Autodesk Fusion 360 part; units mm, degrees
note: some values were not read from the file. Set by a fixed rule: which sketch regions a step uses.
(part 2 of 3)
  constraint symmetric L0.start L152 L410.end
  constraint symmetric L5.start L152 L362.start
  constraint symmetric L6.end L152 L402.end
  constraint symmetric L9.end L152 L528.start
  constraint symmetric L7.end L152 L540.end
  constraint symmetric L18.start L152 L532.start
  constraint symmetric L21.start L152 L528.end
  constraint symmetric L19.start L152 L342.start
  constraint symmetric L9.start L152 L532.end
  constraint symmetric L1.end L152 L522.end
  constraint symmetric L11.end L152 L536.start
  constraint symmetric L1.start L152 L522.start
  constraint symmetric L20.end L152 L529.end
  constraint symmetric L4.start L152 L342.end
  constraint symmetric L4.end L152 L356.end
  constraint symmetric L2.start L152 L336.start
  constraint symmetric L25.start L152 L413.start
  constraint symmetric L24.start L152 L403.end
  constraint symmetric L24.end L152 L420.start
  constraint symmetric L25.end L152 L403.start
  constraint symmetric L29.start L152 L451.end
  constraint symmetric L28.start L152 L405.start
  constraint symmetric L28.end L152 L405.end
  constraint symmetric L29.end L152 L464.start
  constraint symmetric L33.start L152 L415.end
  constraint symmetric L32.start L152 L314.end
  constraint symmetric L32.end L152 L363.end
  constraint symmetric L33.end L152 L314.start
  constraint symmetric L42.start L152 L525.start
  constraint symmetric L49.start L152 L433.end
  constraint symmetric L39.start L152 L423.end
  constraint symmetric L61.start L152 L422.start
  constraint symmetric L57.start L152 L406.start
  constraint symmetric L52.start L152 L422.end
  constraint symmetric L60.end L152 L427.end
  constraint symmetric L52.end L152 L521.end
  constraint symmetric L66.end L152 L524.end
  constraint symmetric L37.end L152 L411.start
  constraint symmetric L47.start L152 L412.end
  constraint symmetric L40.end L152 L441.end
  constraint symmetric L38.end L152 L434.start
  constraint symmetric L40.start L152 L434.end
  constraint symmetric L38.start L152 L443.end
  constraint symmetric L53.end L152 L526.start
  constraint symmetric L48.start L152 L424.start
  constraint symmetric L48.end L152 L424.end
  constraint symmetric L42.end L152 L525.end
  constraint symmetric L50.end L152 L523.end
  constraint symmetric L37.start L152 L416.start
  constraint symmetric L45.start L152 L527.end
  constraint symmetric L58.start L152 L411.end
  constraint symmetric L41.end L152 L407.end
  constraint symmetric L54.end L152 L429.start
  constraint symmetric L41.start L152 L407.start
  constraint symmetric L56.start L152 L533.start
  constraint symmetric L69.end L152 L409.end
  constraint symmetric L36.end L152 L418.start
  constraint symmetric L36.start L152 L425.end
  constraint symmetric L46.end L152 L409.start
  constraint symmetric L44.start L152 L423.start
  constraint symmetric L62.start L152 L526.end
  constraint symmetric L57.end L152 L406.end
  constraint symmetric L39.end L152 L428.end
  constraint symmetric L59.end L152 L534.end
  constraint symmetric L72.start L152 L447.end
  constraint symmetric L73.end L152 L414.start
  constraint symmetric L74.start L152 L414.end
  constraint symmetric L72.end L152 L463.start
  constraint symmetric L79.end L152 L419.end
  constraint symmetric L107.start L152 L312.start
  constraint symmetric L88.start L152 L322.start
  constraint symmetric L91.end L152 L328.start
  constraint symmetric L77.start L152 L324.end
  constraint symmetric L77.end L152 L548.start
  constraint symmetric L78.start L152 L326.start
  constraint symmetric L76.end L152 L330.end
  constraint symmetric L82.end L152 L329.start
  constraint symmetric L84.start L152 L321.start
  constraint symmetric L95.end L152 L323.start
  constraint symmetric L110.end L152 L421.end
  constraint symmetric L83.start L152 L331.start
  constraint symmetric L89.start L152 L327.start
  constraint symmetric L86.end L152 L340.start
  constraint symmetric L98.end L152 L404.end
  constraint symmetric L108.start L152 L310.end
  constraint symmetric L94.end L152 L320.end
  constraint symmetric L113.start L152 L313.end
  constraint symmetric L94.start L152 L320.start
  constraint symmetric L95.start L152 L333.start
  constraint symmetric L81.start L152 L322.end
  constraint symmetric L103.start L152 L315.end
  constraint symmetric L108.end L152 L313.start
  constraint symmetric L82.start L152 L325.end
  constraint symmetric L89.end L152 L327.end
  constraint symmetric L102.end L152 L426.end
  constraint symmetric L84.end L152 L321.end
  constraint symmetric L98.start L152 L312.end
  constraint symmetric L104.start L152 L431.start
  constraint symmetric L103.end L152 L440.end
  constraint symmetric L83.end L152 L331.end
  constraint symmetric L92.end L152 L339.end
  constraint symmetric L105.end L152 L315.start
  constraint symmetric L105.start L152 L471.start
  constraint symmetric L81.end L152 L335.end
  constraint symmetric L92.start L152 L339.start
  constraint symmetric L113.end L152 L310.start
  constraint symmetric L80.start L152 L324.start
  constraint symmetric L76.start L152 L326.end
  constraint symmetric L118.end L152 L318.end
  constraint symmetric L130.end L152 L316.end
  constraint symmetric L147.start L152 L347.start
  constraint symmetric L118.start L152 L318.start
  constraint symmetric L119.end L152 L352.end
  constraint symmetric L134.start L152 L504.end
  constraint symmetric L116.start L152 L511.end
  constraint symmetric L136.start L152 L319.start
  constraint symmetric L136.end L152 L317.start
  constraint symmetric L129.start L152 L311.end
  constraint symmetric L126.start L152 L503.start
  constraint symmetric L130.start L152 L316.start
  constraint symmetric L128.start L152 L317.end
  constraint symmetric L124.start L152 L456.end
  constraint symmetric L124.end L152 L454.start
  constraint symmetric L139.end L152 L364.start
  constraint symmetric L122.start L152 L347.end
  constraint symmetric L119.start L152 L352.start
  constraint symmetric L133.start L152 L359.start
  constraint symmetric L135.end L152 L504.start
  constraint symmetric L116.end L152 L502.start
  constraint symmetric L134.end L152 L511.start
  constraint symmetric L127.start L152 L438.start
  constraint symmetric L143.start L152 L502.end
  constraint symmetric L117.start L152 L344.start
  constraint symmetric L117.end L152 L344.end
  constraint symmetric L121.start L152 L510.end
  constraint symmetric L132.start L152 L462.end
  constraint symmetric L121.end L152 L518.start
  constraint symmetric L123.end L152 L510.start
  constraint symmetric L123.start L152 L438.end
  constraint symmetric L128.end L152 L311.start
  constraint symmetric L133.end L152 L357.start
  constraint symmetric L120.end L152 L346.end
  constraint symmetric L120.start L152 L346.start
  constraint symmetric L125.start L152 L353.end
  constraint symmetric L152 L221.end L442.start
  constraint symmetric L152 L223.start L442.end
  constraint symmetric L152 L222.start L459.end
  constraint symmetric L152 L221.start L460.end
  constraint symmetric L152 L249.start L479.end
  constraint symmetric L152 L231.end L479.start
  constraint symmetric L152 L230.start L488.start
  constraint symmetric L152 L230.end L481.start
  constraint symmetric L152 L226.end L351.start
  constraint symmetric L152 L239.end L380.start
  constraint symmetric L152 L227.start L376.start
  constraint symmetric L152 L235.start L384.end
  constraint symmetric L152 L241.end L387.start
  constraint symmetric L152 L244.start L374.start
  constraint symmetric L152 L242.end L348.start
  constraint symmetric L152 L241.start L487.end
  constraint symmetric L152 L251.end L379.end
  constraint symmetric L152 L238.start L378.end
  constraint symmetric L152 L236.end L368.start
  constraint symmetric L152 L235.end L484.end
  constraint symmetric L152 L234.start L351.end
  constraint symmetric L152 L238.end L379.start
  constraint symmetric L152 L239.start L374.end
  constraint symmetric L152 L243.end L380.end
  constraint symmetric L152 L225.end L383.start
  constraint symmetric L152 L245.start L384.start
  constraint symmetric L152 L250.end L478.start
  constraint symmetric L152 L237.end L368.end
  constraint symmetric L152 L229.end L475.end
  constraint symmetric L152 L225.start L391.start
  constraint symmetric L152 L227.end L376.end
  constraint symmetric L152 L234.end L390.end
  constraint symmetric L152 L229.start L375.end
  constraint symmetric L152 L228.start L398.start
  constraint symmetric L152 L232.start L375.start
  constraint symmetric L152 L228.end L394.start
  constraint symmetric L152 L255.start L348.end
  constraint symmetric L152 L236.start L393.end
  constraint symmetric L152 L231.start L493.end
  constraint symmetric L152 L240.start L486.end
  constraint symmetric L152 L272.start L354.end
  constraint symmetric L152 L274.start L370.end
  constraint symmetric L152 L274.end L386.end
  constraint symmetric L152 L280.start L366.end
  constraint symmetric L152 L283.end L369.end
  constraint symmetric L152 L281.start L373.end
  constraint symmetric L152 L278.end L439.end
  constraint symmetric L152 L276.start L397.end
  constraint symmetric L152 L281.end L366.start
  constraint symmetric L152 L263.end L381.start
  constraint symmetric L152 L289.start L373.start
  constraint symmetric L152 L270.end L477.start
  constraint symmetric L152 L268.end L489.end
  constraint symmetric L152 L276.end L439.start
  constraint symmetric L152 L264.end L349.start
  constraint symmetric L152 L267.end L349.end
  constraint symmetric L152 L261.start L350.start
  constraint symmetric L152 L261.end L350.end
  constraint symmetric L152 L277.end L369.start
  constraint symmetric L152 L279.end L450.end
  constraint symmetric L152 L285.start L457.start
  constraint symmetric L152 L282.end L452.end
  constraint symmetric L152 L266.start L367.start
  constraint symmetric L152 L284.start L457.end
  constraint symmetric L152 L264.start L385.start
  constraint symmetric L152 L275.end L445.start
  constraint symmetric L152 L265.start L476.start
  constraint symmetric L152 L284.end L465.start
  constraint symmetric L152 L286.end L448.start
  constraint symmetric L152 L275.start L446.start
  constraint symmetric L152 L269.end L483.start
  constraint symmetric L152 L269.start L494.start
  constraint symmetric L152 L262.end L371.start
  constraint symmetric L152 L268.start L477.end
  constraint symmetric L152 L262.start L445.end
  constraint symmetric L152 L271.end L371.end
  constraint symmetric L152 P1 P8
  constraint symmetric L152 L298.start L455.start
  constraint symmetric L152 L298.end L455.end
  constraint symmetric L152 P2 P11
  constraint symmetric L152 L299.start L449.start
  constraint symmetric L152 L299.end L449.end
  constraint symmetric L152 P3 P10
  constraint symmetric L152 P4 P9
  constraint symmetric L152 P5 P7
  constraint symmetric L152 P6 P12
  constraint symmetric L152 L305.start L372.start
  constraint symmetric L152 L305.end L372.end
  constraint symmetric L152 L306.start L499.start
  constraint symmetric L152 L306.end L495.start
  constraint symmetric L152 L307.end L495.end
  constraint symmetric L152 L308.start L377.start
  constraint symmetric L152 L308.end L345.start
  constraint symmetric L152 L309.end L345.end
  constraint parallel L8 L550
  constraint perpendicular L550 L551
  constraint perpendicular L551 L552
  constraint tangent L552 A0
  constraint tangent A0 L553
  constraint parallel L285 L553
  constraint coincident L31 L552.end
  constraint coincident L290 A0.start
  constraint coincident L77 L550.end
  constraint symmetric L152 L550.start L554.start
  constraint symmetric L152 L550.end L554.end
  constraint symmetric L152 L551.end L555.end
  constraint symmetric L152 L552.end A1.start
  constraint symmetric L152 A0.start A1.end
  constraint symmetric L152 A0 A1
  constraint symmetric L152 L553.end L557.end
  constraint tangent L550 A2
  constraint tangent L554 A2
  constraint tangent A0 A3
  constraint coincident A3.end L558
  constraint tangent A3 L558
  constraint symmetric L152 A3.end A4.start
  constraint symmetric L152 A3 A4
  measures "d2" distance of L4.start L4.end
  measures "d3" distance of L20.end L4.end
  measures "d6" distance of L9.end L21.start
  measures "d7" distance of L18.start L21.start
  measures "d9" distance of L13.start L8.end
  measures "d10" distance of L13.start L2.start
  measures "d11" distance of L7.end L1.end
  measures "d12" distance of L7.end L11.end
  measures "d13" distance of L15 L17
  measures "d14" distance of L3.start L0.start
  measures "d15" distance of L0.end L0.start
  measures "d16" distance of L6.start L10.end
  measures "d17" distance of L6.start L6.end
  measures "d128" distance of L25.start L24.end
  measures "d129" distance of L25.start L25.end
  measures "d130" distance of L29.start L28.end
  measures "d131" distance of L29.start L29.end
  measures "d132" distance of L9 L11
  measures "d133" distance of L4 L13
  measures "d134" distance of L10 L21
  measures "d135" distance of L5 L22
  measures "d136" distance of L6 L24
  measures "d137" distance of L25 L28
  measures "d138" distance of L33.start L32.end
  measures "d139" distance of L33.start L33.end
  measures "d140" distance of L0 L32
  measures "d141" distance of L1 L8
  measures "d142" distance of L50.end L41.end
  measures "d143" distance of L50.end L45.start
  measures "d144" distance of L56.start L59.end
  measures "d145" distance of L42.start L56.start
  measures "d146" distance of L52.start L52.end
  measures "d147" distance of L52.end L54.end
  measures "d148" distance of L53.end L62.start
  measures "d149" distance of L48.start L62.start
  measures "d150" distance of L48 L52
  measures "d151" distance of L39.start L39.end
  measures "d152" distance of L49.start L39.end
  measures "d153" distance of L57.start L66.end
  measures "d154" distance of L57.start L57.end
  measures "d155" distance of L47.start L37.start
  measures "d156" distance of L37.end L37.start
  measures "d157" distance of L40.end L40.start
  measures "d158" distance of L40.end L38.start
  measures "d159" distance of L59 L62
  measures "d160" distance of L50 L54
  measures "d161" distance of L56 L66
  measures "d162" distance of L44 L45
  measures "d163" distance of L57 L58
  measures "d164" distance of L37 L51
  measures "d165" distance of L36.end L36.start
  measures "d166" distance of L36.end L46.end
  measures "d167" distance of L55 L71
  measures "d169" distance of L7 L67
  measures "d170" distance of L72.start L74.start
  measures "d171" distance of L72.start L72.end
  measures "d172" distance of L46 L75
  measures "d173" distance of L8 L61
  measures "d176" distance of L76.end L76.start
  measures "d177" distance of L79.end L76.end
  measures "d180" distance of L91.end L80.start
  measures "d181" distance of L77.start L80.start
  measures "d191" distance of L78 L80
  measures "d201" distance of L83.start L83.end
  measures "d202" distance of L89.start L83.end
  measures "d203" distance of L86.end L81.end
  measures "d204" distance of L88.start L86.end
  measures "d205" distance of L84.start L84.end
  measures "d206" distance of L82.start L84.end
  measures "d207" distance of L95.end L95.start
  measures "d208" distance of L95.end L94.start
  measures "d209" distance of L84 L94
  measures "d210" distance of L110.end L98.end
  measures "d211" distance of L107.start L110.end
  measures "d212" distance of L102.end L92.end
  measures "d213" distance of L102.end L104.start
  measures "d214" distance of L113.start L113.end
  measures "d215" distance of L108.start L113.end
  measures "d218" distance of L81 L100
  measures "d219" distance of L83 L93
  measures "d220" distance of L90 L92
  measures "d221" distance of L89 L98
  measures "d222" distance of L106 L114
  measures "d224" distance of L103.start L103.end
  measures "d225" distance of L103.end L105.start
  measures "d226" distance of L109 L111
  measures "d227" distance of L82 L96
  measures "d232" distance of L2 L95
  measures "d234" distance of L8 L85
  measures "d235" distance of L8 L91
  measures "d236" distance of L136.end L128.start
  measures "d237" distance of L136.start L136.end
  measures "d238" distance of L136.start L143.start
  measures "d239" distance of L129.start L128.end
  measures "d240" distance of L124.end L139.end
  measures "d241" distance of L119.end L119.start
  measures "d242" distance of L147.start L122.start
  measures "d245" distance of L135.end L121.end
  measures "d246" distance of L117.start L125.start
  measures "d247" distance of L134.start L135.end
  measures "d248" distance of L123.end L123.start
  measures "d249" distance of L127.start L123.start
  measures "d250" distance of L127 L142
  measures "d251" distance of L116.end L143.start
  measures "d252" distance of L138 L151
  measures "d254" distance of L116.start L134.end
  measures "d255" distance of L121.start L123.end
  measures "d256" distance of L129.start L126.start
  measures "d257" distance of L118.end L118.start
  measures "d258" distance of L79 L123
  measures "d261" distance of L155.end L155.start
  measures "d262" distance of L159.end L155.start
  measures "d263" distance of L159.end L159.start
  measures "d264" distance of L157.end L157.start
  measures "d265" distance of L181.start L179.start
  measures "d266" distance of L180.end L182.end
  measures "d267" distance of L180.start L179.end
  measures "d268" distance of L154.end L154.start
  measures "d269" distance of L174.end L171.start
  measures "d270" distance of L153.start L154.end
  measures "d271" distance of L162.end L156.end
  measures "d272" distance of L156.start L156.end
  measures "d273" distance of L156 L187
  measures "d274" distance of L159.start L161.end
  measures "d275" distance of L158 L163
  measures "d276" distance of L158.end L153.end
  measures "d277" distance of L162.end L168.end
  measures "d278" distance of L157.end L165.end
  measures "d279" distance of L167.start L167.end
  measures "d280" distance of L190.end L189.end
  measures "d281" distance of L190.end L191.end
  measures "d282" distance of L194.start L195.end
  measures "d283" distance of L193.start L194.start
  measures "d284" distance of L192 L196
  measures "d285" distance of L187 L194
  measures "d286" distance of P0 L196
  measures "d287" distance of L200.start L197.end
  measures "d288" distance of L200.end L200.start
  measures "d289" distance of L198.start L198.end
  measures "d290" distance of L198.end L199.start
  measures "d291" distance of L198 L203
  measures "d292" distance of L205.end L207.end
  measures "d293" distance of L206.start L207.end
  measures "d294" distance of L202 L206
  measures "d295" distance of L212.end L214.end
  measures "d296" distance of L216.start L214.end
  measures "d297" distance of L217.start L215.end
  measures "d298" distance of L217.end L217.start
  measures "d300" distance of L210.end L209.start
  measures "d301" distance of L209.end L209.start
  measures "d303" distance of L200 L212
  measures "d305" distance of L156 L197
  measures "d306" distance of L221.end L221.start
  measures "d307" distance of L221.end L223.start
  measures "d312" distance of L242.end L237.end
  measures "d313" distance of L236.end L237.end
  measures "d314" distance of L236.end L236.start
  measures "d315" distance of L238.start L255.start
  measures "d316" distance of L241.end L244.start
  measures "d317" distance of L243.end L250.end
  measures "d318" distance of L239.end L239.start
  measures "d319" distance of L230.end L225.start
  measures "d320" distance of L229.start L232.start
  measures "d321" distance of L225.end L225.start
  measures "d322" distance of L249.start L231.end
  measures "d323" distance of L231.end L231.start
  measures "d324" distance of L231 L245
  measures "d325" distance of L234.end L236.start
  measures "d326" distance of L248 L256
  measures "d327" distance of L226.end L234.start
  measures "d328" distance of L249.start L230.start
  measures "d329" distance of L238.start L238.end
  measures "d330" distance of L251.end L245.start
  measures "d375" distance of L272.start L267.end
  measures "d376" distance of L264.end L267.end
  measures "d377" distance of L264.end L264.start
  measures "d378" distance of L261.start L266.start
  measures "d379" distance of L274.start L274.end
  measures "d380" distance of L276.start L276.end
  measures "d381" distance of L283.end L277.end
  measures "d382" distance of L269.end L269.start
  measures "d383" distance of L284.start L284.end
  measures "d384" distance of L270.end L269.end
  measures "d385" distance of L262.end L262.start
  measures "d386" distance of L275.end L262.start
  measures "d387" distance of L289 L290
  measures "d388" distance of L264.start L265.start
  measures "d389" distance of L265 L268
  measures "d390" distance of L268.end L268.start
  measures "d391" distance of L262.end L271.end
  measures "d392" distance of L261.start L261.end
  measures "d393" distance of L263.end L289.start
  measures "d395" distance of origin L220
  measures "d397" angle of L190 L297
  measures "d398" angle of L77 L297
  measures "d399" angle of L30 L221
  measures "d401" distance of L221 L298
  measures "d402" distance of L30 P2
  measures "d403" distance of L29 P2
  measures "d404" distance of L298 P2
  measures "d405" distance of L223 L299
  measures "d406" distance of L77.end L189.end
  measures "d407" angle of L223 L233
  measures "d408" distance of L231 P5
  measures "d409" distance of L240 P5
  measures "d410" distance of L299 P5
  measures "d411" distance of L231 P6
  measures "d412" distance of L260 P6
  measures "d413" distance of L289 L305
  measures "d414" distance of P6 L305
  measures "d415" distance of L127 L306
  measures "d416" distance of L132 L307
  measures "d418" angle of L248 L289
  measures "d419" distance of L289 L308
  measures "d420" distance of L293 L309
  measures "d421" distance of L307 L308.end
  measures "d423" distance of L8 L550
  measures "d424" distance of L63 L551
  measures "d425" distance of L43 L552
extrude "Extrusion10" add sketch "Skizze1" along normal blind 3 makes body 1
sketch "Skizze5" plane through (0, 0, 0) normal (1, 0, 0) x (0, 1, 0)
  line L0 (0, 13.3887) -> (160, 20.3745)
  line L1 (0, 1.75) -> (0, 22.5)
  line L2 (1.75, 0) -> (22.5, 0)
  point P0 (14, 14)
  dimension "d440" = 2.5
  dimension "d441" = 160
  dimension "d450" = 14
  dimension "d451" = 14
  constraint coincident L0.start L1
  constraint coincident L0 P0
  measures "d440" angle of L0 L2
  measures "d441" distance of L0.end L1
  measures "d450" distance of L1 P0
  measures "d451" distance of L2 P0
ref_plane "Arbeitsebene1" through (0, 80, 16.8816) normal (0, 0.043619, -0.999048) x (0, 0.999048, 0.043619)
sketch "Skizze4" plane through (0, 0, 3) normal (0, 0, 1) x (-1, 0, 0)
  line L0 (88.256, -100.8256) -> (90.6871, -87.0383)
  line L1 (90.6871, -87.0383) -> (104.4744, -89.4694)
  line L2 (104.4744, -89.4694) -> (102.0433, -103.2567)
  line L3 (102.0433, -103.2567) -> (88.256, -100.8256)
  line L4 (123.6691, -90.3154) -> (121.238, -104.1027)
  line L5 (121.238, -104.1027) -> (107.4507, -101.6716)
  line L6 (107.4507, -101.6716) -> (109.8818, -87.8843)
  line L7 (109.8818, -87.8843) -> (123.6691, -90.3154)
  line L8 (87.3791, -105.7989) -> (101.1664, -108.23)
  line L9 (101.1664, -108.23) -> (98.7353, -122.0173)
  line L10 (98.7353, -122.0173) -> (84.948, -119.5862)
  line L11 (84.948, -119.5862) -> (87.3791, -105.7989)
  line L12 (100.8347, -139.1928) -> (103.2658, -125.4055)
  line L13 (103.2658, -125.4055) -> (117.0531, -127.8365)
  line L14 (117.0531, -127.8365) -> (114.622, -141.6239)
  line L15 (114.622, -141.6239) -> (100.8347, -139.1928)
  line L16 (97.8584, -126.9906) -> (95.4273, -140.7779)
  line L17 (95.4273, -140.7779) -> (81.64, -138.3468)
  line L18 (81.64, -138.3468) -> (84.0711, -124.5595)
  line L19 (84.0711, -124.5595) -> (97.8584, -126.9906)
  line L20 (-12.05, -83.05) -> (-26.05, -83.05)
  line L21 (-26.05, -83.05) -> (-26.05, -69.05)
  line L22 (-26.05, -69.05) -> (-12.05, -69.05)
  line L23 (-12.05, -69.05) -> (-12.05, -83.05)
  line L24 (147.396, -65.4579) -> (133.6087, -63.0268)
  line L25 (133.6087, -63.0268) -> (136.0398, -49.2395)
  line L26 (136.0398, -49.2395) -> (149.8271, -51.6706)
  line L27 (149.8271, -51.6706) -> (147.396, -65.4579)
  line L28 (29.7949, -103.261) -> (32.226, -89.4737)
  line L29 (32.226, -89.4737) -> (46.0133, -91.9047)
  line L30 (46.0133, -91.9047) -> (43.5823, -105.692)
  line L31 (43.5823, -105.692) -> (29.7949, -103.261)
  line L32 (69.0526, -100.0289) -> (82.8399, -102.46)
  line L33 (82.8399, -102.46) -> (80.4088, -116.2473)
  line L34 (80.4088, -116.2473) -> (66.6215, -113.8162)
  line L35 (66.6215, -113.8162) -> (69.0526, -100.0289)
  line L36 (47.3313, -113.5119) -> (61.1186, -115.9429)
  line L37 (61.1186, -115.9429) -> (58.6875, -129.7302)
  line L38 (58.6875, -129.7302) -> (44.9002, -127.2992)
  line L39 (44.9002, -127.2992) -> (47.3313, -113.5119)
  line L40 (42.7053, -110.6653) -> (40.2743, -124.4526)
  line L41 (40.2743, -124.4526) -> (26.4869, -122.0216)
  line L42 (26.4869, -122.0216) -> (28.918, -108.2342)
  line L43 (28.918, -108.2342) -> (42.7053, -110.6653)
  line L44 (65.7446, -118.7895) -> (79.5319, -121.2205)
  line L45 (79.5319, -121.2205) -> (77.1008, -135.0079)
  line L46 (77.1008, -135.0079) -> (63.3135, -132.5768)
  line L47 (63.3135, -132.5768) -> (65.7446, -118.7895)
  line L48 (48.2082, -108.5386) -> (50.6393, -94.7513)
  line L49 (50.6393, -94.7513) -> (64.4266, -97.1823)
  line L50 (64.4266, -97.1823) -> (61.9955, -110.9697)
  line L51 (61.9955, -110.9697) -> (48.2082, -108.5386)
  line L52 (72.3606, -81.2683) -> (86.1479, -83.6994)
  line L53 (86.1479, -83.6994) -> (83.7168, -97.4867)
  line L54 (83.7168, -97.4867) -> (69.9295, -95.0556)
  line L55 (69.9295, -95.0556) -> (72.3606, -81.2683)
  line L56 (53.9473, -75.9907) -> (67.7346, -78.4218)
  line L57 (67.7346, -78.4218) -> (65.3035, -92.2091)
  line L58 (65.3035, -92.2091) -> (51.5162, -89.778)
  line L59 (51.5162, -89.778) -> (53.9473, -75.9907)
  line L60 (57.2553, -57.2301) -> (71.0426, -59.6612)
  line L61 (71.0426, -59.6612) -> (68.6115, -73.4485)
  line L62 (68.6115, -73.4485) -> (54.8242, -71.0174)
  line L63 (54.8242, -71.0174) -> (57.2553, -57.2301)
  line L64 (75.6686, -62.5077) -> (89.4559, -64.9388)
  line L65 (89.4559, -64.9388) -> (87.0248, -78.7261)
  line L66 (87.0248, -78.7261) -> (73.2375, -76.295)
  line L67 (73.2375, -76.295) -> (75.6686, -62.5077)
  line L68 (46.8808, -85.6605) -> (40.6913, -84.5691)
  line L69 (40.6913, -84.5691) -> (40.548, -85.3816)
  line L70 (40.548, -85.3816) -> (37.8053, -84.898)
  line L71 (37.8053, -84.898) -> (37.9486, -84.0855)
  line L72 (37.9486, -84.0855) -> (34.7677, -83.5246)
  line L73 (34.7677, -83.5246) -> (35.9398, -76.8772)
  line L74 (35.9398, -76.8772) -> (39.1207, -77.4381)
  line L75 (39.1207, -77.4381) -> (39.3855, -75.9362)
  line L76 (39.3855, -75.9362) -> (34.7569, -75.1201)
  line L77 (34.7569, -75.1201) -> (37.188, -61.3328)
  line L78 (37.188, -61.3328) -> (41.8166, -62.1489)
  line L79 (41.8166, -62.1489) -> (42.0814, -60.6471)
  line L80 (42.0814, -60.6471) -> (38.9005, -60.0862)
  line L81 (38.9005, -60.0862) -> (40.0726, -53.4388)
  line L82 (40.0726, -53.4388) -> (43.2536, -53.9996)
  line L83 (43.2536, -53.9996) -> (43.3968, -53.1872)
  line L84 (43.3968, -53.1872) -> (46.1395, -53.6708)
  line L85 (46.1395, -53.6708) -> (45.9962, -54.4833)
  line L86 (45.9962, -54.4833) -> (52.1858, -55.5746)
  line L87 (52.1858, -55.5746) -> (51.8862, -57.2734)
  line L88 (51.8862, -57.2734) -> (53.068, -57.4818)
  line L89 (53.068, -57.4818) -> (52.4949, -60.7317)
  line L90 (52.4949, -60.7317) -> (51.3132, -60.5233)
  line L91 (51.3132, -60.5233) -> (51.0136, -62.2221)
  line L92 (51.0136, -62.2221) -> (46.6115, -61.4459)
  line L93 (46.6115, -61.4459) -> (46.3467, -62.9477)
  line L94 (46.3467, -62.9477) -> (50.9753, -63.7639)
  line L95 (50.9753, -63.7639) -> (48.5442, -77.5512)
  line L96 (48.5442, -77.5512) -> (43.9157, -76.735)
  line L97 (43.9157, -76.735) -> (43.6508, -78.2368)
  line L98 (43.6508, -78.2368) -> (48.0529, -79.0131)
  line L99 (48.0529, -79.0131) -> (47.7534, -80.7118)
  line L100 (47.7534, -80.7118) -> (48.9352, -80.9202)
  line L101 (48.9352, -80.9202) -> (48.3621, -84.1701)
  line L102 (48.3621, -84.1701) -> (47.1803, -83.9617)
  line L103 (47.1803, -83.9617) -> (46.8808, -85.6605)
  line L104 (12.05, -69.05) -> (26.05, -69.05)
  line L105 (26.05, -69.05) -> (26.05, -83.05)
  line L106 (26.05, -83.05) -> (12.05, -83.05)
  line L107 (12.05, -83.05) -> (12.05, -69.05)
  line L108 (26.05, -50) -> (26.05, -64)
  line L109 (26.05, -64) -> (12.05, -64)
  line L110 (12.05, -64) -> (12.05, -50)
  line L111 (12.05, -50) -> (26.05, -50)
  line L112 (-12.05, -50) -> (-12.05, -64)
  line L113 (-12.05, -64) -> (-26.05, -64)
  line L114 (-26.05, -64) -> (-26.05, -50)
  line L115 (-26.05, -50) -> (-12.05, -50)
  line L116 (-7, -50) -> (7, -50)
  line L117 (7, -50) -> (7, -64)
  line L118 (7, -64) -> (-7, -64)
  line L119 (-7, -64) -> (-7, -50)
  line L120 (100.3693, -38.0507) -> (113.525, -42.8389)
  line L121 (113.525, -42.8389) -> (108.7367, -55.9946)
  line L122 (108.7367, -55.9946) -> (95.581, -51.2064)
  line L123 (95.581, -51.2064) -> (100.3693, -38.0507)
  line L124 (69.7598, -36.262) -> (72.1098, -32.1916)
  line L125 (72.1098, -32.1916) -> (84.2342, -39.1916)
  line L126 (84.2342, -39.1916) -> (81.8842, -43.262)
  line L127 (81.8842, -43.262) -> (83.2049, -44.0245)
  line L128 (83.2049, -44.0245) -> (84.8199, -41.2272)
  line L129 (84.8199, -41.2272) -> (90.6655, -44.6022)
  line L130 (90.6655, -44.6022) -> (89.0505, -47.3995)
  line L131 (89.0505, -47.3995) -> (89.765, -47.812)
  line L132 (89.765, -47.812) -> (88.3725, -50.2238)
  line L133 (88.3725, -50.2238) -> (87.658, -49.8113)
  line L134 (87.658, -49.8113) -> (84.5155, -55.2543)
  line L135 (84.5155, -55.2543) -> (83.0216, -54.3918)
  line L136 (83.0216, -54.3918) -> (82.4216, -55.431)
  line L137 (82.4216, -55.431) -> (79.5638, -53.781)
  line L138 (79.5638, -53.781) -> (80.1638, -52.7418)
  line L139 (80.1638, -52.7418) -> (78.6699, -51.8793)
  line L140 (78.6699, -51.8793) -> (80.9049, -48.0082)
  line L141 (80.9049, -48.0082) -> (79.5842, -47.2457)
  line L142 (79.5842, -47.2457) -> (77.2342, -51.316)
  line L143 (77.2342, -51.316) -> (65.1098, -44.316)
  line L144 (65.1098, -44.316) -> (67.4598, -40.2457)
  line L145 (67.4598, -40.2457) -> (66.1391, -39.4832)
  line L146 (66.1391, -39.4832) -> (63.9041, -43.3543)
  line L147 (63.9041, -43.3543) -> (62.4102, -42.4918)
  line L148 (62.4102, -42.4918) -> (61.8102, -43.531)
  line L149 (61.8102, -43.531) -> (58.9523, -41.881)
  line L150 (58.9523, -41.881) -> (59.5523, -40.8418)
  line L151 (59.5523, -40.8418) -> (58.0585, -39.9793)
  line L152 (58.0585, -39.9793) -> (61.201, -34.5363)
  line L153 (61.201, -34.5363) -> (60.4865, -34.1238)
  line L154 (60.4865, -34.1238) -> (61.879, -31.712)
  line L155 (61.879, -31.712) -> (62.5935, -32.1245)
  line L156 (62.5935, -32.1245) -> (64.2085, -29.3272)
  line L157 (64.2085, -29.3272) -> (70.0541, -32.7022)
  line L158 (70.0541, -32.7022) -> (68.4391, -35.4995)
  line L159 (68.4391, -35.4995) -> (69.7598, -36.262)
  line L160 (-65.7446, -118.7895) -> (-63.3135, -132.5768)
  line L161 (-63.3135, -132.5768) -> (-77.1008, -135.0079)
  line L162 (-77.1008, -135.0079) -> (-79.5319, -121.2205)
  line L163 (-79.5319, -121.2205) -> (-65.7446, -118.7895)
  line L164 (-81.64, -138.3468) -> (-95.4273, -140.7779)
  line L165 (-95.4273, -140.7779) -> (-97.8584, -126.9906)
  line L166 (-97.8584, -126.9906) -> (-84.0711, -124.5595)
  line L167 (-84.0711, -124.5595) -> (-81.64, -138.3468)
  line L168 (15.275, -92.8) -> (16.1, -92.8)
  line L169 (16.1, -92.8) -> (16.1, -95.585)
  line L170 (16.1, -95.585) -> (15.275, -95.585)
  line L171 (15.275, -95.585) -> (15.275, -101.87)
  line L172 (15.275, -101.87) -> (13.55, -101.87)
  line L173 (13.55, -101.87) -> (13.55, -103.07)
  line L174 (13.55, -103.07) -> (10.25, -103.07)
  line L175 (10.25, -103.07) -> (10.25, -101.87)
  line L176 (10.25, -101.87) -> (8.525, -101.87)
  line L177 (8.525, -101.87) -> (8.525, -97.4)
  line L178 (8.525, -97.4) -> (7, -97.4)
  line L179 (7, -97.4) -> (7, -102.1)
  line L180 (7, -102.1) -> (-7, -102.1)
  line L181 (-7, -102.1) -> (-7, -97.4)
  line L182 (-7, -97.4) -> (-8.525, -97.4)
  line L183 (-8.525, -97.4) -> (-8.525, -101.87)
  line L184 (-8.525, -101.87) -> (-10.25, -101.87)
  line L185 (-10.25, -101.87) -> (-10.25, -103.07)
  line L186 (-10.25, -103.07) -> (-13.55, -103.07)
  line L187 (-13.55, -103.07) -> (-13.55, -101.87)
  line L188 (-13.55, -101.87) -> (-15.275, -101.87)
  line L189 (-15.275, -101.87) -> (-15.275, -95.585)
  line L190 (-15.275, -95.585) -> (-16.1, -95.585)
  line L191 (-16.1, -95.585) -> (-16.1, -92.8)
  line L192 (-16.1, -92.8) -> (-15.275, -92.8)
  line L193 (-15.275, -92.8) -> (-15.275, -89.57)
  line L194 (-15.275, -89.57) -> (-8.525, -89.57)
  line L195 (-8.525, -89.57) -> (-8.525, -92.8)
  line L196 (-8.525, -92.8) -> (-7, -92.8)
  line L197 (-7, -92.8) -> (-7, -88.1)
  line L198 (-7, -88.1) -> (7, -88.1)
  line L199 (7, -88.1) -> (7, -92.8)
  line L200 (7, -92.8) -> (8.525, -92.8)
  line L201 (8.525, -92.8) -> (8.525, -89.57)
  line L202 (8.525, -89.57) -> (15.275, -89.57)
  line L203 (15.275, -89.57) -> (15.275, -92.8)
  line L204 (-7, -83.05) -> (-7, -69.05)
  line L205 (-7, -69.05) -> (7, -69.05)
  line L206 (7, -69.05) -> (7, -83.05)
  line L207 (7, -83.05) -> (-7, -83.05)
  line L208 (-2.525, -107.15) -> (-2.525, -121.15)
  line L209 (-2.525, -121.15) -> (-16.525, -121.15)
  line L210 (-16.525, -121.15) -> (-16.525, -107.15)
  line L211 (-16.525, -107.15) -> (-2.525, -107.15)
  line L212 (2.525, -121.15) -> (2.525, -107.15)
  line L213 (2.525, -107.15) -> (16.525, -107.15)
  line L214 (16.525, -107.15) -> (16.525, -121.15)
  line L215 (16.525, -121.15) -> (2.525, -121.15)
  line L216 (-46.0133, -91.9047) -> (-32.226, -89.4737)
  line L217 (-32.226, -89.4737) -> (-29.7949, -103.261)
  line L218 (-29.7949, -103.261) -> (-43.5823, -105.692)
  line L219 (-43.5823, -105.692) -> (-46.0133, -91.9047)
  line L220 (-113.1898, -69.1237) -> (-110.7587, -82.911)
  line L221 (-110.7587, -82.911) -> (-124.546, -85.3421)
  line L222 (-124.546, -85.3421) -> (-126.9771, -71.5548)
  line L223 (-126.9771, -71.5548) -> (-113.1898, -69.1237)
  line L224 (-130.3007, -81.7874) -> (-144.088, -84.2185)
  line L225 (-144.088, -84.2185) -> (-146.5191, -70.4311)
  line L226 (-146.5191, -70.4311) -> (-132.7318, -68.0001)
  line L227 (-132.7318, -68.0001) -> (-130.3007, -81.7874)
  line L228 (-149.0613, -85.0954) -> (-162.8486, -87.5265)
  line L229 (-162.8486, -87.5265) -> (-165.2797, -73.7391)
  line L230 (-165.2797, -73.7391) -> (-151.4924, -71.3081)
  line L231 (-151.4924, -71.3081) -> (-149.0613, -85.0954)
  line L232 (-143.2111, -89.1917) -> (-129.4238, -86.7607)
  line L233 (-129.4238, -86.7607) -> (-126.9927, -100.548)
  line L234 (-126.9927, -100.548) -> (-140.78, -102.979)
  line L235 (-140.78, -102.979) -> (-143.2111, -89.1917)
  line L236 (-168.5877, -54.9786) -> (-154.8004, -52.5475)
  line L237 (-154.8004, -52.5475) -> (-152.3693, -66.3348)
  line L238 (-152.3693, -66.3348) -> (-166.1566, -68.7659)
  line L239 (-166.1566, -68.7659) -> (-168.5877, -54.9786)
  line L240 (-147.396, -65.4579) -> (-149.8271, -51.6706)
  line L241 (-149.8271, -51.6706) -> (-136.0398, -49.2395)
  line L242 (-136.0398, -49.2395) -> (-133.6087, -63.0268)
  line L243 (-133.6087, -63.0268) -> (-147.396, -65.4579)
  line L244 (34.0551, -40.0943) -> (34.5854, -39.4624)
  line L245 (34.5854, -39.4624) -> (32.1111, -37.3861)
  line L246 (32.1111, -37.3861) -> (36.4499, -32.2153)
  line L247 (36.4499, -32.2153) -> (38.9242, -34.2916)
  line L248 (38.9242, -34.2916) -> (39.9045, -33.1233)
  line L249 (39.9045, -33.1233) -> (36.3041, -30.1022)
  line L250 (36.3041, -30.1022) -> (45.3031, -19.3776)
  line L251 (45.3031, -19.3776) -> (48.9035, -22.3987)
  line L252 (48.9035, -22.3987) -> (49.8838, -21.2305)
  line L253 (49.8838, -21.2305) -> (47.4094, -19.1543)
  line L254 (47.4094, -19.1543) -> (51.7483, -13.9835)
  line L255 (51.7483, -13.9835) -> (54.2226, -16.0597)
  line L256 (54.2226, -16.0597) -> (54.7529, -15.4277)
  line L257 (54.7529, -15.4277) -> (56.8863, -17.2179)
  line L258 (56.8863, -17.2179) -> (56.356, -17.8499)
  line L259 (56.356, -17.8499) -> (61.1706, -21.8898)
  line L260 (61.1706, -21.8898) -> (60.0618, -23.2112)
  line L261 (60.0618, -23.2112) -> (60.9811, -23.9825)
  line L262 (60.9811, -23.9825) -> (58.8599, -26.5105)
  line L263 (58.8599, -26.5105) -> (57.9406, -25.7392)
  line L264 (57.9406, -25.7392) -> (56.8318, -27.0606)
  line L265 (56.8318, -27.0606) -> (53.4076, -24.1873)
  line L266 (53.4076, -24.1873) -> (52.4273, -25.3555)
  line L267 (52.4273, -25.3555) -> (56.0277, -28.3766)
  line L268 (56.0277, -28.3766) -> (47.0287, -39.1013)
  line L269 (47.0287, -39.1013) -> (43.4283, -36.0802)
  line L270 (43.4283, -36.0802) -> (42.448, -37.2484)
  line L271 (42.448, -37.2484) -> (45.8723, -40.1216)
  line L272 (45.8723, -40.1216) -> (44.7635, -41.4431)
  line L273 (44.7635, -41.4431) -> (45.6827, -42.2144)
  line L274 (45.6827, -42.2144) -> (43.5615, -44.7424)
  line L275 (43.5615, -44.7424) -> (42.6423, -43.971)
  line L276 (42.6423, -43.971) -> (41.5335, -45.2924)
  line L277 (41.5335, -45.2924) -> (36.7189, -41.2525)
  line L278 (36.7189, -41.2525) -> (36.1886, -41.8845)
  line L279 (36.1886, -41.8845) -> (34.0551, -40.0943)
  line L280 (-66.6215, -113.8162) -> (-80.4088, -116.2473)
  line L281 (-80.4088, -116.2473) -> (-82.8399, -102.46)
  line L282 (-82.8399, -102.46) -> (-69.0526, -100.0289)
  line L283 (-69.0526, -100.0289) -> (-66.6215, -113.8162)
  line L284 (-61.1186, -115.9429) -> (-47.3313, -113.5119)
  line L285 (-47.3313, -113.5119) -> (-44.9002, -127.2992)
  line L286 (-44.9002, -127.2992) -> (-58.6875, -129.7302)
  line L287 (-58.6875, -129.7302) -> (-61.1186, -115.9429)
  line L288 (-48.2082, -108.5386) -> (-61.9955, -110.9697)
  line L289 (-61.9955, -110.9697) -> (-64.4266, -97.1823)
  line L290 (-64.4266, -97.1823) -> (-50.6393, -94.7513)
  line L291 (-50.6393, -94.7513) -> (-48.2082, -108.5386)
  line L292 (-127.854, -66.5815) -> (-130.2851, -52.7942)
  line L293 (-130.2851, -52.7942) -> (-116.4978, -50.3631)
  line L294 (-116.4978, -50.3631) -> (-114.0667, -64.1504)
  line L295 (-114.0667, -64.1504) -> (-127.854, -66.5815)
  line L296 (-95.581, -51.2064) -> (-108.7367, -55.9946)
  line L297 (-108.7367, -55.9946) -> (-113.525, -42.8389)
  line L298 (-113.525, -42.8389) -> (-100.3693, -38.0507)
  line L299 (-100.3693, -38.0507) -> (-95.581, -51.2064)
  line L300 (-68.6115, -73.4485) -> (-71.0426, -59.6612)
  line L301 (-71.0426, -59.6612) -> (-57.2553, -57.2301)
  line L302 (-57.2553, -57.2301) -> (-54.8242, -71.0174)
  line L303 (-54.8242, -71.0174) -> (-68.6115, -73.4485)
  line L304 (-81.8842, -43.262) -> (-84.2342, -39.1916)
  line L305 (-84.2342, -39.1916) -> (-72.1098, -32.1916)
  line L306 (-72.1098, -32.1916) -> (-69.7598, -36.262)
  line L307 (-69.7598, -36.262) -> (-68.4391, -35.4995)
  line L308 (-68.4391, -35.4995) -> (-70.0541, -32.7022)
  line L309 (-70.0541, -32.7022) -> (-64.2085, -29.3272)
  line L310 (-64.2085, -29.3272) -> (-62.5935, -32.1245)
  line L311 (-62.5935, -32.1245) -> (-61.879, -31.712)
  line L312 (-61.879, -31.712) -> (-60.4865, -34.1238)
  line L313 (-60.4865, -34.1238) -> (-61.201, -34.5363)
  line L314 (-61.201, -34.5363) -> (-58.0585, -39.9793)
  line L315 (-58.0585, -39.9793) -> (-59.5523, -40.8418)
  line L316 (-59.5523, -40.8418) -> (-58.9523, -41.881)
  line L317 (-58.9523, -41.881) -> (-61.8102, -43.531)
  line L318 (-61.8102, -43.531) -> (-62.4102, -42.4918)
  line L319 (-62.4102, -42.4918) -> (-63.9041, -43.3543)
  line L320 (-63.9041, -43.3543) -> (-66.1391, -39.4832)
  line L321 (-66.1391, -39.4832) -> (-67.4598, -40.2457)
  line L322 (-67.4598, -40.2457) -> (-65.1098, -44.316)
  line L323 (-65.1098, -44.316) -> (-77.2342, -51.316)
  line L324 (-77.2342, -51.316) -> (-79.5842, -47.2457)
  line L325 (-79.5842, -47.2457) -> (-80.9049, -48.0082)
  line L326 (-80.9049, -48.0082) -> (-78.6699, -51.8793)
  line L327 (-78.6699, -51.8793) -> (-80.1638, -52.7418)
  line L328 (-80.1638, -52.7418) -> (-79.5638, -53.781)
  line L329 (-79.5638, -53.781) -> (-82.4216, -55.431)
  line L330 (-82.4216, -55.431) -> (-83.0216, -54.3918)
  line L331 (-83.0216, -54.3918) -> (-84.5155, -55.2543)
  line L332 (-84.5155, -55.2543) -> (-87.658, -49.8113)
  line L333 (-87.658, -49.8113) -> (-88.3725, -50.2238)
  line L334 (-88.3725, -50.2238) -> (-89.765, -47.812)
  line L335 (-89.765, -47.812) -> (-89.0505, -47.3995)
  line L336 (-89.0505, -47.3995) -> (-90.6655, -44.6022)
  line L337 (-90.6655, -44.6022) -> (-84.8199, -41.2272)
  line L338 (-84.8199, -41.2272) -> (-83.2049, -44.0245)
  line L339 (-83.2049, -44.0245) -> (-81.8842, -43.262)
  line L340 (-39.3855, -75.9362) -> (-39.1207, -77.4381)
  line L341 (-39.1207, -77.4381) -> (-35.9398, -76.8772)
  line L342 (-35.9398, -76.8772) -> (-34.7677, -83.5246)
  line L343 (-34.7677, -83.5246) -> (-37.9486, -84.0855)
  line L344 (-37.9486, -84.0855) -> (-37.8053, -84.898)
  line L345 (-37.8053, -84.898) -> (-40.548, -85.3816)
  line L346 (-40.548, -85.3816) -> (-40.6913, -84.5691)
  line L347 (-40.6913, -84.5691) -> (-46.8808, -85.6605)
  line L348 (-46.8808, -85.6605) -> (-47.1803, -83.9617)
  line L349 (-47.1803, -83.9617) -> (-48.3621, -84.1701)
  line L350 (-48.3621, -84.1701) -> (-48.9352, -80.9202)
  line L351 (-48.9352, -80.9202) -> (-47.7534, -80.7118)
  line L352 (-47.7534, -80.7118) -> (-48.0529, -79.0131)
  line L353 (-48.0529, -79.0131) -> (-43.6508, -78.2368)
  line L354 (-43.6508, -78.2368) -> (-43.9157, -76.735)
  line L355 (-43.9157, -76.735) -> (-48.5442, -77.5512)
  line L356 (-48.5442, -77.5512) -> (-50.9753, -63.7639)
  line L357 (-50.9753, -63.7639) -> (-46.3467, -62.9477)
  line L358 (-46.3467, -62.9477) -> (-46.6115, -61.4459)
  line L359 (-46.6115, -61.4459) -> (-51.0136, -62.2221)
  line L360 (-51.0136, -62.2221) -> (-51.3132, -60.5233)
  line L361 (-51.3132, -60.5233) -> (-52.4949, -60.7317)
  line L362 (-52.4949, -60.7317) -> (-53.068, -57.4818)
  line L363 (-53.068, -57.4818) -> (-51.8862, -57.2734)
  line L364 (-51.8862, -57.2734) -> (-52.1858, -55.5746)
  line L365 (-52.1858, -55.5746) -> (-45.9962, -54.4833)
  line L366 (-45.9962, -54.4833) -> (-46.1395, -53.6708)
  line L367 (-46.1395, -53.6708) -> (-43.3968, -53.1872)
  line L368 (-43.3968, -53.1872) -> (-43.2536, -53.9996)
  line L369 (-43.2536, -53.9996) -> (-40.0726, -53.4388)
  line L370 (-40.0726, -53.4388) -> (-38.9005, -60.0862)
  line L371 (-38.9005, -60.0862) -> (-42.0814, -60.6471)
  line L372 (-42.0814, -60.6471) -> (-41.8166, -62.1489)
  line L373 (-41.8166, -62.1489) -> (-37.188, -61.3328)
  line L374 (-37.188, -61.3328) -> (-34.7569, -75.1201)
  line L375 (-34.7569, -75.1201) -> (-39.3855, -75.9362)
  line L376 (-42.7053, -110.6653) -> (-28.918, -108.2342)
  line L377 (-28.918, -108.2342) -> (-26.4869, -122.0216)
  line L378 (-26.4869, -122.0216) -> (-40.2743, -124.4526)
  line L379 (-40.2743, -124.4526) -> (-42.7053, -110.6653)
  line L380 (-114.622, -141.6239) -> (-117.0531, -127.8365)
  line L381 (-117.0531, -127.8365) -> (-103.2658, -125.4055)
  line L382 (-103.2658, -125.4055) -> (-100.8347, -139.1928)
  line L383 (-100.8347, -139.1928) -> (-114.622, -141.6239)
  line L384 (-106.5738, -106.6449) -> (-104.1427, -120.4322)
  line L385 (-104.1427, -120.4322) -> (-117.93, -122.8633)
  line L386 (-117.93, -122.8633) -> (-120.3611, -109.076)
  line L387 (-120.3611, -109.076) -> (-106.5738, -106.6449)
  line L388 (-152.9246, -143.8082) -> (-155.3557, -130.0209)
  line L389 (-155.3557, -130.0209) -> (-141.5684, -127.5898)
  line L390 (-141.5684, -127.5898) -> (-139.1373, -141.3771)
  line L391 (-139.1373, -141.3771) -> (-152.9246, -143.8082)
  line L392 (-105.3513, -84.4961) -> (-107.7824, -70.7088)
  line L393 (-107.7824, -70.7088) -> (-93.9951, -68.2777)
  line L394 (-93.9951, -68.2777) -> (-91.564, -82.065)
  line L395 (-91.564, -82.065) -> (-105.3513, -84.4961)
  line L396 (-102.0433, -103.2567) -> (-104.4744, -89.4694)
  line L397 (-104.4744, -89.4694) -> (-90.6871, -87.0383)
  line L398 (-90.6871, -87.0383) -> (-88.256, -100.8256)
  line L399 (-88.256, -100.8256) -> (-102.0433, -103.2567)
  line L400 (-142.4453, -122.6166) -> (-156.2326, -125.0476)
  line L401 (-156.2326, -125.0476) -> (-158.6637, -111.2603)
  line L402 (-158.6637, -111.2603) -> (-144.8764, -108.8292)
  line L403 (-144.8764, -108.8292) -> (-142.4453, -122.6166)
  line L404 (-39.9045, -33.1233) -> (-38.9242, -34.2916)
  line L405 (-38.9242, -34.2916) -> (-36.4499, -32.2153)
  line L406 (-36.4499, -32.2153) -> (-32.1111, -37.3861)
  line L407 (-32.1111, -37.3861) -> (-34.5854, -39.4624)
  line L408 (-34.5854, -39.4624) -> (-34.0551, -40.0943)
  line L409 (-34.0551, -40.0943) -> (-36.1886, -41.8845)
  line L410 (-36.1886, -41.8845) -> (-36.7189, -41.2525)
  line L411 (-36.7189, -41.2525) -> (-41.5335, -45.2924)
  line L412 (-41.5335, -45.2924) -> (-42.6423, -43.971)
  line L413 (-42.6423, -43.971) -> (-43.5615, -44.7424)
  line L414 (-43.5615, -44.7424) -> (-45.6827, -42.2144)
  line L415 (-45.6827, -42.2144) -> (-44.7635, -41.4431)
  line L416 (-44.7635, -41.4431) -> (-45.8723, -40.1216)
  line L417 (-45.8723, -40.1216) -> (-42.448, -37.2484)
  line L418 (-42.448, -37.2484) -> (-43.4283, -36.0802)
  line L419 (-43.4283, -36.0802) -> (-47.0287, -39.1013)
  line L420 (-47.0287, -39.1013) -> (-56.0277, -28.3766)
  line L421 (-56.0277, -28.3766) -> (-52.4273, -25.3555)
  line L422 (-52.4273, -25.3555) -> (-53.4076, -24.1873)
  line L423 (-53.4076, -24.1873) -> (-56.8318, -27.0606)
  line L424 (-56.8318, -27.0606) -> (-57.9406, -25.7392)
  line L425 (-57.9406, -25.7392) -> (-58.8599, -26.5105)
  line L426 (-58.8599, -26.5105) -> (-60.9811, -23.9825)
  line L427 (-60.9811, -23.9825) -> (-60.0618, -23.2112)
  line L428 (-60.0618, -23.2112) -> (-61.1706, -21.8898)
  line L429 (-61.1706, -21.8898) -> (-56.356, -17.8499)
  line L430 (-56.356, -17.8499) -> (-56.8863, -17.2179)
  line L431 (-56.8863, -17.2179) -> (-54.7529, -15.4277)
  line L432 (-54.7529, -15.4277) -> (-54.2226, -16.0597)
  line L433 (-54.2226, -16.0597) -> (-51.7483, -13.9835)
  line L434 (-51.7483, -13.9835) -> (-47.4094, -19.1543)
  line L435 (-47.4094, -19.1543) -> (-49.8838, -21.2305)
  line L436 (-49.8838, -21.2305) -> (-48.9035, -22.3987)
  line L437 (-48.9035, -22.3987) -> (-45.3031, -19.3776)
  line L438 (-45.3031, -19.3776) -> (-36.3041, -30.1022)
  line L439 (-36.3041, -30.1022) -> (-39.9045, -33.1233)
  line L440 (-65.3035, -92.2091) -> (-67.7346, -78.4218)
  line L441 (-67.7346, -78.4218) -> (-53.9473, -75.9907)
  line L442 (-53.9473, -75.9907) -> (-51.5162, -89.778)
  line L443 (-51.5162, -89.778) -> (-65.3035, -92.2091)
  line L444 (-89.4559, -64.9388) -> (-75.6686, -62.5077)
  line L445 (-75.6686, -62.5077) -> (-73.2375, -76.295)
  line L446 (-73.2375, -76.295) -> (-87.0248, -78.7261)
  line L447 (-87.0248, -78.7261) -> (-89.4559, -64.9388)
  line L448 (-83.7168, -97.4867) -> (-86.1479, -83.6994)
  line L449 (-86.1479, -83.6994) -> (-72.3606, -81.2683)
  line L450 (-72.3606, -81.2683) -> (-69.9295, -95.0556)
  line L451 (-69.9295, -95.0556) -> (-83.7168, -97.4867)
  line L452 (-107.4507, -101.6716) -> (-121.238, -104.1027)
  line L453 (-121.238, -104.1027) -> (-123.6691, -90.3154)
  line L454 (-123.6691, -90.3154) -> (-109.8818, -87.8843)
  line L455 (-109.8818, -87.8843) -> (-107.4507, -101.6716)
  line L456 (-145.7533, -103.856) -> (-159.5406, -106.287)
  line L457 (-159.5406, -106.287) -> (-161.9717, -92.4997)
  line L458 (-161.9717, -92.4997) -> (-148.1844, -90.0687)
  line L459 (-148.1844, -90.0687) -> (-145.7533, -103.856)
  line L460 (-137.472, -121.7396) -> (-139.9031, -107.9523)
  line L461 (-139.9031, -107.9523) -> (-126.1158, -105.5212)
  line L462 (-126.1158, -105.5212) -> (-123.6847, -119.3086)
  line L463 (-123.6847, -119.3086) -> (-137.472, -121.7396)
  line L464 (-98.7353, -122.0173) -> (-101.1664, -108.23)
  line L465 (-101.1664, -108.23) -> (-87.3791, -105.7989)
  line L466 (-87.3791, -105.7989) -> (-84.948, -119.5862)
  line L467 (-84.948, -119.5862) -> (-98.7353, -122.0173)
  line L468 (-134.164, -140.5002) -> (-136.5951, -126.7129)
  line L469 (-136.5951, -126.7129) -> (-122.8078, -124.2818)
  line L470 (-122.8078, -124.2818) -> (-120.3767, -138.0691)
  line L471 (-120.3767, -138.0691) -> (-134.164, -140.5002)
  line L472 (144.088, -84.2185) -> (130.3007, -81.7874)
  line L473 (130.3007, -81.7874) -> (132.7318, -68.0001)
  line L474 (132.7318, -68.0001) -> (146.5191, -70.4311)
  line L475 (146.5191, -70.4311) -> (144.088, -84.2185)
  line L476 (120.3611, -109.076) -> (117.93, -122.8633)
  line L477 (117.93, -122.8633) -> (104.1427, -120.4322)
  line L478 (104.1427, -120.4322) -> (106.5738, -106.6449)
  line L479 (106.5738, -106.6449) -> (120.3611, -109.076)
  line L480 (126.9771, -71.5548) -> (124.546, -85.3421)
  line L481 (124.546, -85.3421) -> (110.7587, -82.911)
  line L482 (110.7587, -82.911) -> (113.1898, -69.1237)
  line L483 (113.1898, -69.1237) -> (126.9771, -71.5548)
  line L484 (161.9717, -92.4997) -> (159.5406, -106.287)
  line L485 (159.5406, -106.287) -> (145.7533, -103.856)
  line L486 (145.7533, -103.856) -> (148.1844, -90.0687)
  line L487 (148.1844, -90.0687) -> (161.9717, -92.4997)
  line L488 (120.3767, -138.0691) -> (122.8078, -124.2818)
  line L489 (122.8078, -124.2818) -> (136.5951, -126.7129)
  line L490 (136.5951, -126.7129) -> (134.164, -140.5002)
  line L491 (134.164, -140.5002) -> (120.3767, -138.0691)